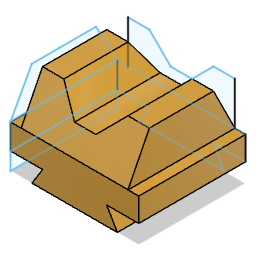
200100_Assignment_1 (Autodesk Fusion 360 design; units mm, degrees)
Autodesk Fusion 360 part; units mm, degrees
sketch "Front View" plane through (0, 0, 0) normal (0, 0, 1) x (1, 0, 0)
  line L0 (0, 19.879) -> (0, 8.1508)
  line L1 (0, 8.1508) -> (15, 8.1508)
  line L2 (15, 8.1508) -> (10, 0.1508)
  line L3 (10, 0.1508) -> (50, 0.1508)
  line L4 (50, 0.1508) -> (45, 8.777)
  line L5 (45, 8.777) -> (60, 8.777)
  line L6 (60, 8.777) -> (60, 19.879)
  line L7 (60, 19.879) -> (0, 19.879)
  line L8 (5, 19.879) -> (5, 39.879)
  line L9 (5, 39.879) -> (15, 39.879)
  line L10 (25, 29.879) -> (35, 29.879)
  line L11 (45, 39.953) -> (55, 39.953)
  line L12 (55, 39.953) -> (55, 19.879)
  line L13 (15, 39.879) -> (25, 29.879)
  line L14 (35, 29.879) -> (45, 39.953)
  dimension "d1" = 8
  dimension "d2" = 11.7282
  dimension "d3" = 10
  dimension "d4" = 40
  dimension "d5" = 30
  dimension "d6" = 20
  dimension "d7" = 60
  dimension "d8" = 5
  dimension "d9" = 5
  dimension "d10" = 10
  dimension "d11" = 10
  dimension "d12" = 10
  dimension "d13" = 10
  dimension "d14" = 10
  dimension "d16" = 10
  dimension "d17" = 5
  constraint vertical L0
  constraint perpendicular L0 L1
  constraint perpendicular L0 L3
  constraint parallel L3 L5
  constraint perpendicular L5 L6
  constraint perpendicular L6 L7
  constraint coincident L7 L8.start
  constraint perpendicular L7 L8
  constraint perpendicular L8 L9
  constraint perpendicular L8 L10
  constraint parallel L10 L11
  constraint coincident L7 L12.end
  constraint perpendicular L7 L12
  measures "d1" vertical distance of L1.end L2.end
  measures "d2" distance of L0.start L0.end
  measures "d3" horizontal distance of origin L2.end
  measures "d4" distance of L2.end L3.end
  measures "d5" horizontal distance of L1.end L4.end
  measures "d6" distance of L8.start L8.end
  measures "d7" distance of L0.start L6.end
  measures "d8" distance of L0.start L8.start
  measures "d9" distance of L6.end L12.end
  measures "d10" distance of L8.end L9.end
  measures "d11" distance of L10.start L10.end
  measures "d12" distance of L11.start L11.end
  measures "d13" horizontal distance of L3.end L5.end
  measures "d14" horizontal distance of L10.start L9.end
  measures "d16" vertical distance of L10.start L9.end
  measures "d17" horizontal distance of L1.end L2.end
extrude "Extrude1" add sketch "Front View" along normal blind 50 contours L0 L1 L2 L3 L4 L5 L6 L7
sketch "Side View" plane through (0, 0, 0) normal (1, 0, 0) x (0, 0, -1)
  line L0 (-50.0346, 20.0445) -> (-40.0346, 38.5513)
  line L1 (-27, 38.5513) -> (-40.0346, 38.5513)
  line L2 (-27, 38.5513) -> (-10.0346, 38.5513)
  line L3 (-0.0346, 20.0445) -> (-10.0346, 38.5513)
  line L4 (-50.0346, 20.0445) -> (-0.0346, 20.0445)
  line L5 (-50.0346, 20.0445) -> (-0.0346, 20.0445)
  line L6 (-0.0346, 20.0445) -> (-0.0346, 8.0445)
  line L7 (-0.0346, 8.0445) -> (-50.0346, 8.0445)
  line L8 (-50.0346, 8.0445) -> (-50.0346, 20.0445)
  line L9 (-50.0346, 8.0445) -> (-0.0346, 8.0445)
  line L10 (-0.0346, 8.0445) -> (-0.0346, 0.0445)
  line L11 (-0.0346, 0.0445) -> (-50.0346, 0.0445)
  line L12 (-50.0346, 0.0445) -> (-50.0346, 8.0445)
  dimension "d32" = 12
  dimension "d33" = 50
  dimension "d34" = 50
  dimension "d35" = 8
  dimension "d36" = 30
  dimension "d37" = 10
  dimension "d38" = 10
  constraint horizontal L1
  constraint parallel L1 L2
  constraint horizontal L4
  constraint horizontal L5
  constraint vertical L6
  constraint horizontal L7
  constraint vertical L8
  constraint horizontal L9
  constraint vertical L10
  constraint horizontal L11
  constraint vertical L12
  measures "d32" distance of L0.start L7.end
  measures "d33" distance of L0.start L3.start
  measures "d34" distance of L7.end L6.end
  measures "d35" distance of L7.end L11.end
  measures "d36" distance of L0.end L2.end
  measures "d37" horizontal distance of L0.start L0.end
  measures "d38" horizontal distance of L2.end L3.start
extrude "Extrude4" add sketch "Front View" along normal blind 50 contours L7 L8 L9 L10 L11 L12 L13 L14
chamfer "Chamfer2" distance 20 distance2 10 1 edges at (50, 39.953, 0) measured on face at (28.3333, 15.6022, 0)
chamfer "Chamfer3" distance 20 distance2 10 1 edges at (50, 39.953, 50) measured on face at (28.3333, 15.6022, 50)
extrude "Extrude3" [suppressed]
named bodies: "200100_AMAN_ASSIGNMENT1"
